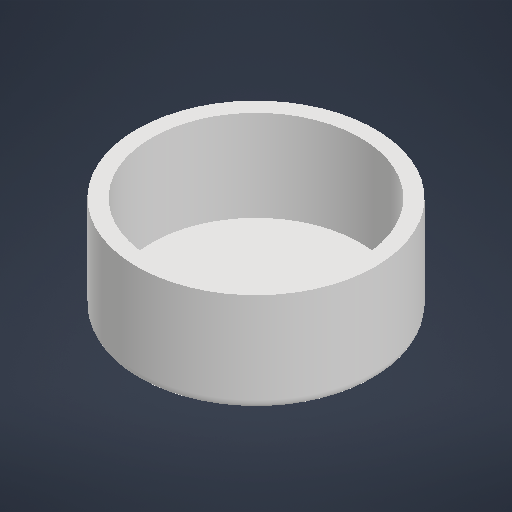
# Autodesk Inventor part: Bottle
Saved by Autodesk Inventor 2026 (Build 300175050, 175E)
## iProperties
Created: 2026-03-25
Part Number: Bottle
Material: Generic
Document SubType Name: Modeling
Designer: sniel
Density: 1 g/cm^3
Appearance: Default
Author: sniel
Autodesk Inventor part; units mm, degrees
ref_plane "YZ Plane" through (0, 0, 0) normal (1, 0, 0) x (0, 1, 0)
ref_plane "XZ Plane" through (0, 0, 0) normal (0, 1, 0) x (-1, 0, 0)
ref_plane "XY Plane" through (0, 0, 0) normal (0, 0, 1) x (1, 0, 0)
sketch "Sketch1" plane through (0, 0, 0) normal (0, 1, 0) x (-1, 0, 0)
  circle A0 centre (0, 0) radius 14.75
  line L0 (0, -14.75) -> (0, -12.9)
  circle A1 centre (0, 0) radius 12.9
  dimension "d0" = 29.5
  dimension "d1" = 1.85
  constraints: 2 coincident, 2 end point, 2 vertical alignment, 1 vertical, 4 other
  measures "d1" distance of L0.start L0.end
extrude "Extrusion1" add sketch "Sketch1" along normal blind 1.2 contours A1 | A0
sketch "Sketch2" plane through (0, 1.2, 0) normal (0, 1, 0) x (1, 0, 0)
  circle A0 centre (0, 0) radius 14.75 projected
  line L0 (0, 14.75) -> (0, 12.9)
  circle A1 centre (0, 0) radius 12.9
  dimension "d4" = 1.85
  constraints: 2 end point, 2 vertical alignment, 1 coincident, 1 vertical, 3 other
  measures "d4" distance of L0.start L0.end
extrude "Extrusion2" add sketch "Sketch2" along normal blind 11.25
fillet "Fillet1" radius 1.2 1 edges at (14.75, 0, 0)
body "Solid1"
